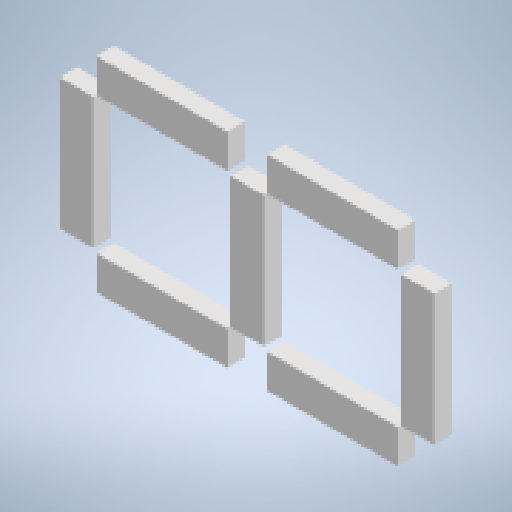
# Autodesk Inventor part: Digit
Saved by Autodesk Inventor 2024.2 (Build 282272000, 272)
## iProperties
Created: 2024-01-22
Part Number: Digit
Material: Generic
Document SubType Name: Modeling
Designer: Felix
Density: 1 g/cm^3
Appearance: Default
Author: Felix
Autodesk Inventor part; units mm, degrees
ref_plane "YZ Plane" through (0, 0, 0) normal (1, 0, 0) x (0, 1, 0)
ref_plane "XZ Plane" through (0, 0, 0) normal (0, 1, 0) x (-1, 0, 0)
ref_plane "XY Plane" through (0, 0, 0) normal (0, 0, 1) x (1, 0, 0)
sketch "Sketch1" plane through (0, 0, 0) normal (0, 1, 0) x (-1, 0, 0)
  line L0 (86, 43) -> (0, 43) construction
  line L1 (0, 43) -> (0, -43) construction
  line L2 (0, -43) -> (86, -43) construction
  line L3 (86, -43) -> (86, 43) construction
  line L4 (0, 43) -> (-86, 43) construction
  line L5 (-86, 43) -> (-86, -43) construction
  line L6 (-86, -43) -> (0, -43) construction
  line L7 (0, -43) -> (0, 43) construction
  line L8 (76, 51.5) -> (10, 51.5)
  line L9 (10, 51.5) -> (10, 34.5)
  line L10 (10, 34.5) -> (76, 34.5)
  line L11 (76, 34.5) -> (76, 51.5)
  line L12 (8.5, 33) -> (-8.5, 33)
  line L13 (-8.5, 33) -> (-8.5, -33)
  line L14 (-8.5, -33) -> (8.5, -33)
  line L15 (8.5, -33) -> (8.5, 33)
  line L16 (86, 0) -> (-86, 0) construction
  line L17 (43, 43) -> (43, -43) construction
  line L18 (77.5, 33) -> (94.5, 33)
  line L19 (94.5, 33) -> (94.5, -33)
  line L20 (94.5, -33) -> (77.5, -33)
  line L21 (77.5, -33) -> (77.5, 33)
  line L22 (-43, 43) -> (-43, -43) construction
  line L23 (-94.5, 33) -> (-77.5, 33)
  line L24 (-77.5, 33) -> (-77.5, -33)
  line L25 (-77.5, -33) -> (-94.5, -33)
  line L26 (-94.5, -33) -> (-94.5, 33)
  line L27 (-76, 51.5) -> (-10, 51.5)
  line L28 (-10, 51.5) -> (-10, 34.5)
  line L29 (-10, 34.5) -> (-76, 34.5)
  line L30 (-76, 34.5) -> (-76, 51.5)
  line L31 (76, -51.5) -> (10, -51.5)
  line L32 (10, -51.5) -> (10, -34.5)
  line L33 (10, -34.5) -> (76, -34.5)
  line L34 (76, -34.5) -> (76, -51.5)
  line L35 (-10, -51.5) -> (-10, -34.5)
  line L36 (-10, -34.5) -> (-76, -34.5)
  line L37 (-76, -51.5) -> (-10, -51.5)
  line L38 (-76, -34.5) -> (-76, -51.5)
  point P0 (0, 0)
  point P1 (0, 0)
  point P2 (76, 43)
  point P3 (0, 33)
  point P4 (86, 33)
  point P5 (-86, 0)
  point P6 (-86, 33)
  point P7 (-76, 43)
  point P8 (76, -43)
  point P9 (-76, -43)
  dimension "d2" = 86
  dimension "d3" = 86
  dimension "d4" = 17
  dimension "d5" = 17
  dimension "d6" = 66
  dimension "d7" = 66
  dimension "d8" = 86
  constraints: 78 end point, 27 symmetric about line, 9 midpoint, 8 parallel, 4 horizontal, 4 perpendicular, 3 coincident, 3 point on line, 2 other
  measures "d2" distance of L2.end L0.start
  measures "d3" distance of L0.end L4.end
  measures "d4" distance of L10.end L8.start
  measures "d5" distance of L12.start L12.end
  measures "d6" distance of L8.start L8.end
  measures "d7" distance of L14.end L12.start
  measures "d8" distance of L0.start L0.end
extrude "Extrusion1" add sketch "Sketch1" along normal blind 9
equation "\"d2\" = d8"
equation "\"d3\" = d8"
equation "\"d5\" = d4"
equation "\"d7\" = d6"
body "Solid1"
